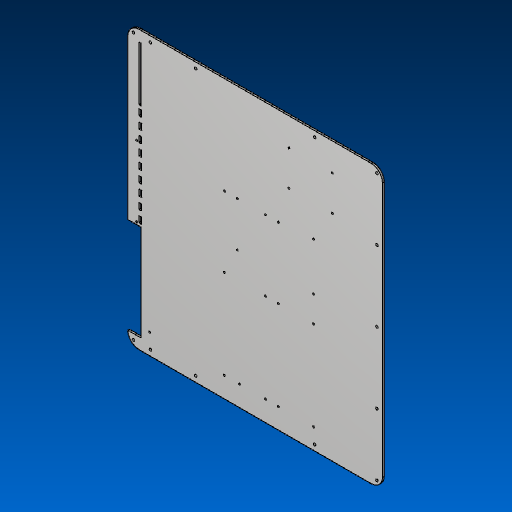
# Autodesk Inventor part: right_panel
Saved by Autodesk Inventor 2018 (Build 220112000, 112)
## iProperties
Created: 2019-10-14
Part Number: right_panel
Material: アルミニウム 6061
Document SubType Name: Modeling
Designer: gisen
Density: 2.7 g/cm^3
Appearance: アルミニウム - フラット
Author: gisen
Autodesk Inventor part; units mm, degrees
ref_plane "YZ Plane" through (0, 0, 0) normal (1, 0, 0) x (0, 1, 0)
ref_plane "XZ Plane" through (0, 0, 0) normal (0, 1, 0) x (-1, 0, 0)
ref_plane "XY Plane" through (0, 0, 0) normal (0, 0, 1) x (1, 0, 0)
sketch "スケッチ1" plane through (0, 0, 0) normal (0, 0, 1) x (1, 0, 0)
  line L0 (-205, -245) -> (205, -245)
  line L1 (225, -225) -> (225, 225)
  line L2 (205, 245) -> (-205, 245)
  line L3 (-225, 225) -> (-225, -225)
  line L4 (-225, -245) -> (225, 245) construction
  line L5 (225, -245) -> (-225, 245) construction
  circle A0 centre (-215, 235) radius 2.25
  circle A1 centre (215, 235) radius 2.25
  circle A2 centre (-215, -235) radius 2.25
  circle A3 centre (215, -235) radius 2.25
  arc A4 (-205, 245) -> (-225, 225) centre (-205, 225) ccw
  arc A5 (225, 225) -> (205, 245) centre (205, 225) ccw
  arc A6 (205, -245) -> (225, -225) centre (205, -225) ccw
  arc A7 (-225, -225) -> (-205, -245) centre (-205, -225) ccw
  point P0 (0, 0)
  dimension "d0" = 450
  dimension "d1" = 490
  dimension "d2" = 4.5
  dimension "d3" = 10
  dimension "d4" = 10
  dimension "d5" = 10
  dimension "d6" = 10
  dimension "d7" = 10
  dimension "d8" = 10
  dimension "d9" = 10
  dimension "d10" = 10
  dimension "d11" = 20
  constraints: 12 end point, 8 centre point, 8 point on circle, 8 point on line, 8 tangent, 6 equal radius, 2 midpoint, 2 parallel, 1 horizontal, 1 perpendicular
  measures "d0" distance of L5.end L4.end
  measures "d1" distance of L4.end L5.start
  measures "d2" diameter of A0
  measures "d3" distance from line of A0.centre L2
  measures "d4" distance from line of L3 A0.centre
  measures "d5" distance from line of A1.centre L2
  measures "d6" distance from line of L1 A1.centre
  measures "d7" distance from line of L1 A3.centre
  measures "d8" distance from line of L0 A3.centre
  measures "d9" distance from line of L0 A2.centre
  measures "d10" distance from line of L3 A2.centre
  measures "d11" radius of A4
extrude "押し出し1" add sketch "スケッチ1" along normal blind 3
sketch "スケッチ2" plane through (0, 0, 3) normal (0, 0, 1) x (1, 0, 0)
  circle A0 centre (18.0923, 72.9265) radius 1.6
  circle A1 centre (-54.2977, 72.9265) radius 1.6
  circle A2 centre (-209.2377, 72.9265) radius 1.6
  circle A3 centre (-209.2377, -51.5335) radius 1.6
  circle A4 centre (-186.3777, -209.0135) radius 1.6
  circle A5 centre (-54.2977, -209.0135) radius 1.6
  circle A6 centre (18.0923, -209.0135) radius 1.6
  circle A7 centre (18.0923, -51.5335) radius 1.6
  circle A8 centre (-54.2977, -51.5335) radius 1.6
  circle A9 centre (38.092, -209.014) radius 2.25 projected
  circle A10 centre (-166.378, -209.014) radius 2.25 projected
  circle A11 centre (38.092, -51.534) radius 2.25 projected
  circle A12 centre (38.092, 72.926) radius 2.25 projected
  circle A13 centre (-34.298, -209.014) radius 2.25 projected
  circle A14 centre (-34.298, -51.534) radius 2.25 projected
  circle A15 centre (-34.298, 72.926) radius 2.25 projected
  circle A16 centre (-189.238, -51.534) radius 2.25 projected
  circle A17 centre (-189.238, 72.926) radius 2.25 projected
  point P0 (0, 0)
  dimension "d14" = 3.2
  constraints: 9 centre point, 8 equal radius
  measures "d14" diameter of A0
extrude "押し出し2" cut sketch "スケッチ2" against normal blind 3 contours A0 | A1 | A2 | A3 | A4 | A5 | A6 | A7 | A8
sketch "スケッチ4" plane through (0, 0, 3) normal (0, 0, 1) x (1, 0, 0)
  line L0 (-205, -225) -> (-202, -225) projected
  line L1 (-205, -50.8937) -> (-205, -40.6067) projected
  line L2 (-205, -50.8937) -> (-202, -50.8937) projected
  line L3 (-202, -40.6067) -> (-202, -50.8937) projected
  line L4 (-205, -40.6067) -> (-202, -40.6067) projected
  line L5 (-205, -30.5483) -> (-205, -20.2613) projected
  line L6 (-205, -30.5483) -> (-202, -30.5483) projected
  line L7 (-202, -20.2613) -> (-202, -30.5483) projected
  line L8 (-205, -20.2613) -> (-202, -20.2613) projected
  line L9 (-205, -9.8937) -> (-205, 0.3933) projected
  line L10 (-205, -9.8937) -> (-202, -9.8937) projected
  line L11 (-202, 0.3933) -> (-202, -9.8937) projected
  line L12 (-205, 0.3933) -> (-202, 0.3933) projected
  line L13 (-205, 10.4517) -> (-205, 20.7387) projected
  line L14 (-205, 10.4517) -> (-202, 10.4517) projected
  line L15 (-202, 20.7387) -> (-202, 10.4517) projected
  line L16 (-205, 20.7387) -> (-202, 20.7387) projected
  line L17 (-205, 31.1063) -> (-205, 41.3933) projected
  line L18 (-205, 31.1063) -> (-202, 31.1063) projected
  line L19 (-202, 41.3933) -> (-202, 31.1063) projected
  line L20 (-205, 41.3933) -> (-202, 41.3933) projected
  line L21 (-205, 51.4517) -> (-205, 61.7387) projected
  line L22 (-205, 51.4517) -> (-202, 51.4517) projected
  line L23 (-202, 61.7387) -> (-202, 51.4517) projected
  line L24 (-205, 61.7387) -> (-202, 61.7387) projected
  line L25 (-205, 72.1063) -> (-205, 82.3933) projected
  line L26 (-205, 72.1063) -> (-202, 72.1063) projected
  line L27 (-202, 82.3933) -> (-202, 72.1063) projected
  line L28 (-205, 82.3933) -> (-202, 82.3933) projected
  line L29 (-205, 92.4517) -> (-205, 102.7387) projected
  line L30 (-205, 92.4517) -> (-202, 92.4517) projected
  line L31 (-202, 102.7387) -> (-202, 92.4517) projected
  line L32 (-205, 102.7387) -> (-202, 102.7387) projected
  line L33 (-205, 225) -> (-205, 129.6) projected
  line L34 (-205, 129.6) -> (-202, 129.6) projected
  line L35 (-202, 225) -> (-202, 129.6) projected
  line L36 (-205, 225) -> (-202, 225) projected
  line L37 (-202, 102.7387) -> (-201, 102.7387)
  line L38 (-201, 102.7387) -> (-201, 92.4517)
  line L39 (-201, 92.4517) -> (-202, 92.4517)
  line L40 (-202, 82.3933) -> (-201, 82.3933)
  line L41 (-201, 82.3933) -> (-201, 72.1063)
  line L42 (-201, 72.1063) -> (-202, 72.1063)
  line L43 (-202, 61.7387) -> (-201, 61.7387)
  line L44 (-201, 61.7387) -> (-201, 51.4517)
  line L45 (-201, 51.4517) -> (-202, 51.4517)
  line L46 (-202, 41.3933) -> (-201, 41.3933)
  line L47 (-201, 41.3933) -> (-201, 31.1063)
  line L48 (-201, 31.1063) -> (-202, 31.1063)
  line L49 (-202, 20.7387) -> (-201, 20.7387)
  line L50 (-201, 20.7387) -> (-201, 10.4517)
  line L51 (-201, 10.4517) -> (-202, 10.4517)
  line L52 (-202, 0.3933) -> (-201, 0.3933)
  line L53 (-201, 0.3933) -> (-201, -9.8937)
  line L54 (-201, -9.8937) -> (-202, -9.8937)
  line L55 (-202, -20.2613) -> (-201, -20.2613)
  line L56 (-201, -20.2613) -> (-201, -30.5483)
  line L57 (-201, -30.5483) -> (-202, -30.5483)
  line L58 (-202, -40.6067) -> (-201, -40.6067)
  line L59 (-201, -40.6067) -> (-201, -50.8937)
  line L60 (-201, -50.8937) -> (-202, -50.8937)
  line L61 (-205, -56.064) -> (-205, -225) projected
  line L62 (-202, -56.064) -> (-202, -225) projected
  line L63 (-205, 112.7971) -> (-202, 112.7971) projected
  line L64 (-205, 123.0841) -> (-205, 112.7971) projected
  line L65 (-205, 123.0841) -> (-202, 123.0841) projected
  line L66 (-202, 112.7971) -> (-201, 112.7971)
  line L67 (-201, 112.7971) -> (-201, 123.0841)
  line L68 (-201, 123.0841) -> (-202, 123.0841)
  line L69 (-205, -56.064) -> (-202, -56.064) projected
  point P0 (0, 0)
  point P1 (-225, -58.3552)
  point P2 (-222, -58.3552)
  point P3 (-225, -120.4005)
  point P4 (-222, -120.4005)
  dimension "d17" = 1
  constraints: 54 end point, 16 perpendicular, 9 equal length, 9 horizontal, 1 collinear, 4 other
  measures "d17" distance of L31.start L37.end
extrude "押し出し3" cut sketch "スケッチ4" against normal blind 3
sketch "スケッチ5" plane through (0, 0, 3) normal (0, 0, 1) x (1, 0, 0)
  circle A0 centre (-215, 235) radius 2.25 construction
  circle A1 centre (-215, -235) radius 2.25 construction
  circle A2 centre (-185, -235) radius 2.25
  line L0 (-205, -245) -> (205, -245) projected
  circle A3 centre (-185, 235) radius 2.25
  line L1 (205, 245) -> (-205, 245) projected
  point P0 (0, 0)
  dimension "d20" = 30
  dimension "d21" = 10
  dimension "d22" = 30
  dimension "d23" = 10
  constraints: 2 centre point, 2 equal radius
  measures "d20" distance of A1.centre A2.centre
  measures "d21" distance from line of L0 A2.centre
  measures "d22" distance of A0.centre A3.centre
  measures "d23" distance from line of L1 A3.centre
extrude "押し出し4" cut sketch "スケッチ5" against normal blind 3
sketch "スケッチ6" plane through (0, 0, 3) normal (0, 0, 1) x (1, 0, 0)
  circle A0 centre (-185, -235) radius 2.25 construction
  circle A1 centre (-185, 235) radius 2.25 construction
  circle A2 centre (18.0923, -51.5335) radius 1.6 construction
  circle A3 centre (-54.2977, -209.0135) radius 1.6 construction
  circle A4 centre (-209.2377, -51.5335) radius 1.6 construction
  circle A5 centre (-54.2977, 72.9265) radius 1.6 construction
  circle A6 centre (18.0923, 72.9265) radius 1.6 construction
  circle A7 centre (-209.2377, 72.9265) radius 1.6 construction
  circle A8 centre (-186.3777, -209.0135) radius 1.6 construction
  circle A9 centre (18.0923, -209.0135) radius 1.6 construction
  circle A10 centre (-54.2977, -51.5335) radius 1.6 construction
  circle A11 centre (215, -235) radius 2.25 construction
  circle A12 centre (-215, -235) radius 2.25 construction
  circle A13 centre (215, 235) radius 2.25 construction
  circle A14 centre (-215, 235) radius 2.25 construction
  line L0 (205, 245) -> (-205, 245) construction
  arc A15 (-205, 245) -> (-225, 225) centre (-205, 225) ccw construction
  line L1 (-225, 225) -> (-225, -225) construction
  arc A16 (-225, -225) -> (-205, -245) centre (-205, -225) ccw construction
  line L2 (-205, -245) -> (205, -245) construction
  arc A17 (205, -245) -> (225, -225) centre (205, -225) ccw construction
  line L3 (225, -225) -> (225, 225) construction
  arc A18 (225, 225) -> (205, 245) centre (205, 225) ccw construction
  line L4 (-201.8, 129.4) -> (-205.2, 129.4)
  line L5 (-205.2, 129.4) -> (-205.2, 225.2)
  line L6 (-205.2, 225.2) -> (-201.8, 225.2)
  line L7 (-201.8, 225.2) -> (-201.8, 129.4)
  line L8 (-200.8, 102.9387) -> (-200.8, 92.2517)
  line L9 (-200.8, 92.2517) -> (-205.2, 92.2517)
  line L10 (-205.2, 92.2517) -> (-205.2, 102.9387)
  line L11 (-205.2, 102.9387) -> (-200.8, 102.9387)
  line L12 (-200.8, 82.5933) -> (-200.8, 71.9063)
  line L13 (-200.8, 71.9063) -> (-205.2, 71.9063)
  line L14 (-205.2, 71.9063) -> (-205.2, 82.5933)
  line L15 (-205.2, 82.5933) -> (-200.8, 82.5933)
  line L16 (-200.8, 61.9387) -> (-200.8, 51.2517)
  line L17 (-200.8, 51.2517) -> (-205.2, 51.2517)
  line L18 (-205.2, 51.2517) -> (-205.2, 61.9387)
  line L19 (-205.2, 61.9387) -> (-200.8, 61.9387)
  line L20 (-200.8, 41.5933) -> (-200.8, 30.9063)
  line L21 (-200.8, 30.9063) -> (-205.2, 30.9063)
  line L22 (-205.2, 30.9063) -> (-205.2, 41.5933)
  line L23 (-205.2, 41.5933) -> (-200.8, 41.5933)
  line L24 (-200.8, 20.9387) -> (-200.8, 10.2517)
  line L25 (-200.8, 10.2517) -> (-205.2, 10.2517)
  line L26 (-205.2, 10.2517) -> (-205.2, 20.9387)
  line L27 (-205.2, 20.9387) -> (-200.8, 20.9387)
  line L28 (-200.8, 0.5933) -> (-200.8, -10.0937)
  line L29 (-200.8, -10.0937) -> (-205.2, -10.0937)
  line L30 (-205.2, -10.0937) -> (-205.2, 0.5933)
  line L31 (-205.2, 0.5933) -> (-200.8, 0.5933)
  line L32 (-200.8, -20.0613) -> (-200.8, -30.7483)
  line L33 (-200.8, -30.7483) -> (-205.2, -30.7483)
  line L34 (-205.2, -30.7483) -> (-205.2, -20.0613)
  line L35 (-205.2, -20.0613) -> (-200.8, -20.0613)
  line L36 (-200.8, -40.4067) -> (-200.8, -51.0937)
  line L37 (-200.8, -51.0937) -> (-205.2, -51.0937)
  line L38 (-205.2, -51.0937) -> (-205.2, -40.4067)
  line L39 (-205.2, -40.4067) -> (-200.8, -40.4067)
  line L40 (-201.8, -55.864) -> (-225.2, -55.864)
  line L41 (-225.2, -55.864) -> (-225.2, -225.2)
  line L42 (-225.2, -225.2) -> (-201.8, -225.2)
  line L43 (-201.8, -225.2) -> (-201.8, -55.864)
  line L44 (-202, -56.064) -> (-202, -225) projected
  line L45 (-205, 0.3933) -> (-201, 0.3933) projected
  line L46 (-201, 0.3933) -> (-201, -9.8937) projected
  line L47 (-201, -9.8937) -> (-205, -9.8937) projected
  line L48 (-205, 102.7387) -> (-201, 102.7387) projected
  line L49 (-201, 102.7387) -> (-201, 92.4517) projected
  line L50 (-201, 92.4517) -> (-205, 92.4517) projected
  line L51 (-205, 82.3933) -> (-201, 82.3933) projected
  line L52 (-201, 82.3933) -> (-201, 72.1063) projected
  line L53 (-201, 72.1063) -> (-205, 72.1063) projected
  line L54 (-205, 61.7387) -> (-201, 61.7387) projected
  line L55 (-201, 61.7387) -> (-201, 51.4517) projected
  line L56 (-201, 51.4517) -> (-205, 51.4517) projected
  line L57 (-205, 41.3933) -> (-201, 41.3933) projected
  line L58 (-201, 41.3933) -> (-201, 31.1063) projected
  line L59 (-201, 31.1063) -> (-205, 31.1063) projected
  line L60 (-205, 20.7387) -> (-201, 20.7387) projected
  line L61 (-201, 20.7387) -> (-201, 10.4517) projected
  line L62 (-201, 10.4517) -> (-205, 10.4517) projected
  line L63 (-205, 225) -> (-202, 225) projected
  line L64 (-202, 129.6) -> (-205, 129.6) projected
  line L65 (-202, -225) -> (-205, -225) projected
  line L66 (-202, 225) -> (-202, 129.6) projected
  line L67 (-201, -30.5483) -> (-205, -30.5483) projected
  line L68 (-205, -20.2613) -> (-201, -20.2613) projected
  line L69 (-201, -20.2613) -> (-201, -30.5483) projected
  line L70 (-201, -50.8937) -> (-205, -50.8937) projected
  line L71 (-205, -40.6067) -> (-201, -40.6067) projected
  line L72 (-200.8, 112.5971) -> (-205.2, 112.5971)
  line L73 (-205.2, 112.5971) -> (-205.2, 123.2841)
  line L74 (-205.2, 123.2841) -> (-200.8, 123.2841)
  line L75 (-200.8, 123.2841) -> (-200.8, 112.5971)
  line L76 (-201, 112.7971) -> (-205, 112.7971) projected
  line L77 (-205, 123.0841) -> (-201, 123.0841) projected
  line L78 (-205, -56.064) -> (-202, -56.064) projected
  line L79 (-205, 123.0841) -> (-201, 123.0841) projected
  line L80 (-201, 123.0841) -> (-201, 112.7971) projected
  line L81 (-201, 112.7971) -> (-205, 112.7971) projected
  line L82 (-205, -40.6067) -> (-201, -40.6067) projected
  line L83 (-201, -40.6067) -> (-201, -50.8937) projected
  line L84 (-201, -50.8937) -> (-205, -50.8937) projected
  line L85 (-205, 129.6) -> (-205, 225) projected
  line L86 (-205, 92.4517) -> (-205, 102.7387) projected
  line L87 (-205, 51.4517) -> (-205, 61.7387) projected
  line L88 (-205, 10.4517) -> (-205, 20.7387) projected
  line L89 (-205, -50.8937) -> (-205, -40.6067) projected
  line L90 (-205, -9.8937) -> (-205, 0.3933) projected
  line L91 (-205, -30.5483) -> (-205, -20.2613) projected
  line L92 (-205, 31.1063) -> (-205, 41.3933) projected
  line L93 (-205, 72.1063) -> (-205, 82.3933) projected
  line L94 (-205, 112.7971) -> (-205, 123.0841) projected
  line L95 (-205, -225) -> (-205, -56.064) projected
  point P0 (0, 0)
  dimension "d78" = 0.2
  dimension "d79" = 0.2
  dimension "d81" = 0.2
  dimension "d82" = 0.2
  dimension "d83" = 0.2
  dimension "d84" = 0.2
  dimension "d85" = 0.2
  dimension "d87" = 0.2
  dimension "d89" = 0.2
  dimension "d90" = 0.2
  dimension "d91" = 0.2
  dimension "d92" = 0.2
  dimension "d93" = 0.2
  dimension "d95" = 0.2
  dimension "d96" = 0.2
  dimension "d97" = 0.2
  dimension "d98" = 0.2
  dimension "d99" = 0.2
  dimension "d100" = 0.2
  dimension "d101" = 0.2
  dimension "d102" = 0.2
  dimension "d103" = 0.2
  constraints: 88 end point, 17 vertical alignment, 16 vertical, 3 horizontal, 2 parallel, 2 perpendicular
  measures "d78" distance between parallel lines of L65 L42
  measures "d79" distance between parallel lines of L44 L43
  measures "d81" distance between parallel lines of L37 L70
  measures "d82" distance between parallel lines of L39 L71
  measures "d83" distance between parallel lines of L33 L67
  measures "d84" distance between parallel lines of L68 L35
  measures "d85" distance between parallel lines of L47 L29
  measures "d87" distance between parallel lines of L62 L25
  measures "d89" distance between parallel lines of L59 L21
  measures "d90" distance between parallel lines of L23 L57
  measures "d91" distance between parallel lines of L56 L17
  measures "d92" distance between parallel lines of L19 L54
  measures "d93" distance between parallel lines of L53 L13
  measures "d95" distance between parallel lines of L50 L9
  measures "d96" distance between parallel lines of L11 L48
  measures "d97" distance between parallel lines of L76 L72
  measures "d98" distance between parallel lines of L74 L77
  measures "d99" distance between parallel lines of L4 L64
  measures "d100" distance between parallel lines of L63 L6
  measures "d101" distance from line of L36 L70.start
  measures "d102" distance from line of L38 L70.end
  measures "d103" distance from line of L7 L64.start
extrude "押し出し5" cut sketch "スケッチ6" against normal through all contours L4 L5 L6 L7 | L8 L9 L10 L11 | L12 L13 L14 L15 | L16 L17 L18 L19 | L20 L21 L22 L23 | L24 L25 L26 L27 | L28 L29 L30 L31 | L32 L33 L34 L35 | L36 L37 L38 L39 | L43 L42 L41 L40 | L44 L65 L95 L78 | L45 L46 L47 L90 | L48 L49 L50 L86 | L51 L52 L53 L93 | L54 L55 L56 L87 | L57 L58 L59 L92 | L60 L61 L62 L88 | L63 L66 L64 L85 | L67 L91 L68 L69 | L70 L89 L71 L83 | L72 L73 L74 L75 | L76 L94 L77 L80
sketch "スケッチ7" plane through (0, 0, 3) normal (0, 0, 1) x (1, 0, 0)
  line L0 (225, 225) -> (225, -225) projected
  circle A0 centre (-105, -235) radius 2.25 projected
  circle A1 centre (215, 0) radius 2.25 projected
  circle A2 centre (105, -235) radius 2.25 projected
  circle A3 centre (215, 125) radius 2.25 projected
  circle A4 centre (-105, 235) radius 2.25 projected
  circle A5 centre (-215, -125) radius 2.25 projected
  circle A6 centre (-215, 0) radius 2.25 projected
  circle A7 centre (105, 235) radius 2.25 projected
  circle A8 centre (215, -125) radius 2.25 projected
  line L1 (-205.2, 132.4) -> (-201.8, 132.4) projected
  line L2 (-201.8, 132.4) -> (-201.8, 225.2) projected
  line L3 (-205.2, 225.2) -> (-201.8, 225.2) projected
  circle A9 centre (215, 235) radius 2.25 projected
  circle A10 centre (-215, 235) radius 2.25 projected
  circle A11 centre (215, -235) radius 2.25 projected
  circle A12 centre (-215, -235) radius 2.25 projected
  line L4 (205, -245) -> (-205, -245) projected
  arc A13 (-225, -225) -> (-205, -245) centre (-205, -225) ccw projected
  line L5 (-225, -225) -> (-225, 225) projected
  arc A14 (-205, 245) -> (-225, 225) centre (-205, 225) ccw projected
  line L6 (-205, 245) -> (205, 245) projected
  arc A15 (225, 225) -> (205, 245) centre (205, 225) ccw projected
  line L7 (225, 225) -> (225, -225) projected
  arc A16 (205, -245) -> (225, -225) centre (205, -225) ccw projected
  line L8 (-205.2, 132.4) -> (-205.2, 225.2) projected
  circle A17 centre (-215, 125) radius 2.25 projected
  point P0 (0, 0)
  point P1 (-212.7501, 124.9816)
  point P2 (-217.2499, 124.9816)
extrude "押し出し6" cut sketch "スケッチ7" against normal up to surface (3 mm away) contours A0 | A1 | A2 | A3 | A4 | A7 | A8
sketch "スケッチ8" plane through (0, 0, 0) normal (0, 0, -1) x (-1, 0, 0)
  line L0 (-49.775, 130.075) -> (-150.225, 130.075) construction
  line L1 (-150.225, 130.075) -> (-150.225, 199.925) construction
  line L2 (-150.225, 199.925) -> (-49.775, 199.925) construction
  line L3 (-49.775, 199.925) -> (-49.775, 130.075) construction
  line L4 (-49.775, 130.075) -> (-150.225, 199.925) construction
  line L5 (-150.225, 130.075) -> (-49.775, 199.925) construction
  line L6 (205, 245) -> (-205, 245) construction
  line L7 (-225, 225) -> (-225, -225) construction
  line L8 (-59.625, 195.86) -> (-136.225, 195.86) construction
  line L9 (-136.225, 195.86) -> (-136.225, 134.14) construction
  line L10 (-136.225, 134.14) -> (-59.625, 134.14) construction
  line L11 (-59.625, 134.14) -> (-59.625, 195.86) construction
  line L12 (-59.625, 195.86) -> (-136.225, 134.14) construction
  line L13 (-136.225, 195.86) -> (-59.625, 134.14) construction
  line L14 (-97.925, 165) -> (-100, 165) construction
  circle A0 centre (-59.625, 134.14) radius 1.6
  circle A1 centre (-59.625, 195.86) radius 1.6
  circle A2 centre (-136.225, 195.86) radius 1.6
  circle A3 centre (-136.225, 134.14) radius 1.6
  point P0 (0, 0)
  dimension "d40" = 69.85
  dimension "d41" = 100.45
  dimension "d42" = 80
  dimension "d43" = 125
  dimension "d44" = 61.72
  dimension "d45" = 90.6
  dimension "d46" = 14
  dimension "d47" = 3.2
  dimension "d48" = 3.2
  dimension "d49" = 3.2
  dimension "d50" = 3.2
  constraints: 26 end point, 4 centre point, 4 coincident, 4 midpoint, 4 parallel, 3 horizontal, 2 perpendicular
  measures "d40" distance of L0.end L1.end
  measures "d41" distance of L0.start L0.end
  measures "d42" distance from line of L6 L14.end
  measures "d43" distance from line of L7 L14.end
  measures "d44" distance of L10.end L8.start
  measures "d45" distance between parallel lines of L1 L11
  measures "d46" distance between parallel lines of L1 L9
  measures "d47" diameter of A0
  measures "d48" diameter of A1
  measures "d49" diameter of A2
  measures "d50" diameter of A3
extrude "押し出し7" cut sketch "スケッチ8" against normal through all
sketch "スケッチ9" plane through (0, 0, 0) normal (0, 0, -1) x (-1, 0, 0)
  circle A0 centre (186.3777, -209.0135) radius 1.6 construction
  circle A1 centre (54.2977, -209.0135) radius 1.6 construction
  circle A2 centre (-18.0923, -209.0135) radius 1.6 construction
  circle A3 centre (209.2377, -51.5335) radius 1.6 construction
  circle A4 centre (209.2377, 72.9265) radius 1.6 construction
  circle A5 centre (54.2977, 72.9265) radius 1.6 construction
  circle A6 centre (-18.0923, 72.9265) radius 1.6 construction
  circle A7 centre (54.2977, -51.5335) radius 1.6 construction
  circle A8 centre (-18.0923, -51.5335) radius 1.6 construction
  line L0 (219.3977, -215.3635) -> (-52.3823, -215.3635) construction
  line L1 (-52.3823, -215.3635) -> (-52.3823, 89.4365) construction
  line L2 (-52.3823, 89.4365) -> (219.3977, 89.4365) construction
  line L3 (219.3977, 89.4365) -> (219.3977, -215.3635) construction
  point P0 (0, 0)
  dimension "d53" = 6.35
  dimension "d54" = 33.02
  dimension "d55" = 304.8
  dimension "d56" = 271.78
  constraints: 8 end point, 2 parallel, 1 horizontal, 1 perpendicular
  measures "d53" distance from line of A0.centre L0
  measures "d54" distance from line of L3 A0.centre
  measures "d55" distance of L2.end L0.start
  measures "d56" distance of L0.start L0.end
sketch "スケッチ10" plane through (0, 0, 0) normal (0, 0, -1) x (-1, 0, 0)
  line L0 (219.3977, -215.3635) -> (-110.8023, -215.3635) construction
  line L1 (-110.8023, -215.3635) -> (-110.8023, 89.4365) construction
  line L2 (-110.8023, 89.4365) -> (219.3977, 89.4365) construction
  line L3 (219.3977, 89.4365) -> (219.3977, -215.3635) construction
  circle A0 centre (209.2377, 72.9265) radius 1.6 construction
  circle A1 centre (-215, -125) radius 2.25 projected
  circle A2 centre (-103.1823, 78.0065) radius 1.6
  circle A3 centre (209.2377, 72.9265) radius 1.6 construction
  line L4 (209.2377, 72.9265) -> (54.2977, 72.9265) construction
  circle A4 centre (54.2977, 72.9265) radius 1.6 construction
  circle A5 centre (54.2977, 72.9265) radius 1.6 construction
  line L5 (54.2977, 72.9265) -> (-18.0923, 72.9265) construction
  line L6 (-18.0923, 72.9265) -> (-40.9523, 72.9265) construction
  circle A6 centre (-18.0923, 72.9265) radius 1.6
  circle A7 centre (-40.9523, 72.9265) radius 1.6
  line L7 (-103.1823, 78.0065) -> (-103.1823, -5.8135) construction
  line L8 (-103.1823, -5.8135) -> (-103.1823, -51.5335) construction
  line L9 (-103.1823, -51.5335) -> (-103.1823, -208.9135) construction
  circle A8 centre (-103.1823, -5.8135) radius 1.6
  circle A9 centre (-103.1823, -51.5335) radius 1.6
  circle A10 centre (-103.1823, -208.9135) radius 1.6
  line L10 (-103.1823, -5.8135) -> (31.4377, -5.8135) construction
  circle A11 centre (31.4377, -5.8135) radius 1.6
  line L11 (31.4377, -5.8135) -> (31.4377, 72.9265) construction
  circle A12 centre (31.4377, 72.9265) radius 1.6
  line L12 (209.2377, 72.9265) -> (209.2377, -209.0135) construction
  circle A13 centre (186.3777, -209.0135) radius 1.6 construction
  line L13 (209.2377, -209.0135) -> (186.3777, -209.0135) construction
  circle A14 centre (209.2377, -209.0135) radius 1.6
  line L14 (-40.9523, 72.9265) -> (-40.9523, -209.0135) construction
  line L15 (-40.9523, -209.0135) -> (-18.0923, -209.0135) construction
  circle A15 centre (-18.0923, -51.5335) radius 1.6 construction
  line L16 (-18.0923, -51.5335) -> (-40.9523, -51.5335) construction
  circle A16 centre (-18.0923, -209.0135) radius 1.6 construction
  circle A17 centre (-40.9523, -51.5335) radius 1.6
  circle A18 centre (-40.9523, -209.0135) radius 1.6
  line L17 (-18.0923, -209.0135) -> (186.3777, -209.0135) construction
  circle A19 centre (27.6277, -209.0135) radius 1.6
  point P0 (0, 0)
  dimension "d57" = 330.2
  dimension "d58" = 304.8
  dimension "d59" = 10.16
  dimension "d60" = 16.51
  dimension "d61" = 104.1977
  dimension "d62" = 5.08
  dimension "d63" = 312.42
  dimension "d64" = 154.94
  dimension "d65" = 227.33
  dimension "d66" = 250.19
  dimension "d67" = 78.74
  dimension "d68" = 124.46
  dimension "d69" = 281.84
  dimension "d70" = 177.8
  dimension "d71" = 134.62
  dimension "d72" = 16.51
  dimension "d73" = 181.61
  dimension "d74" = 3.2
  constraints: 36 end point, 14 centre point, 13 coincident, 13 equal radius, 6 point on line, 5 horizontal, 4 perpendicular, 4 vertical, 2 parallel
  measures "d57" distance of L0.start L0.end
  measures "d58" distance of L0.end L1.end
  measures "d59" distance from line of A0.centre L3
  measures "d60" distance from line of L2 A0.centre
  measures "d61" distance from line of L1 A1.centre
  measures "d62" vertical distance of A0.centre L7.start
  measures "d63" horizontal distance of A0.centre L7.start
  measures "d64" distance of L4.start L4.end
  measures "d65" distance of L5.end L4.start
  measures "d66" distance of L4.start L6.end
  measures "d67" vertical distance of L10.start A0.centre
  measures "d68" vertical distance of L8.end A0.centre
  measures "d69" vertical distance of L4.start L9.end
  measures "d70" horizontal distance of L4.start L10.end
  measures "d71" distance of L10.start L10.end
  measures "d72" distance from line of L2 L11.end
  measures "d73" distance from line of L12 A19.centre
  measures "d74" diameter of A0
extrude "押し出し8" cut sketch "スケッチ10" against normal blind 10 contours A2 | A7 | A8 | A9 | A10 | A11 | A12 | A14 | A17 | A18 | A19
equation "\"d5\" = d3"
equation "\"d6\" = d4"
equation "\"d7\" = d6"
equation "\"d8\" = d5"
equation "\"d9\" = d8"
equation "\"d10\" = d7"
